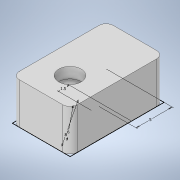
# Autodesk Inventor part: Bearing_Differential
Saved by Autodesk Inventor 2022.1 (Build 261234020, 234B)
## iProperties
Created: 2022-08-27
Part Number: Bearing_Differential
Material: Generic
Document SubType Name: Modeling
Designer: cdug029
Density: 1 g/cm^3
Appearance: Default
Author: cdug029
Autodesk Inventor part; units mm, degrees
ref_plane "YZ Plane" through (0, 0, 0) normal (1, 0, 0) x (0, 1, 0)
ref_plane "XZ Plane" through (0, 0, 0) normal (0, 1, 0) x (-1, 0, 0)
ref_plane "XY Plane" through (0, 0, 0) normal (0, 0, 1) x (1, 0, 0)
sketch "Sketch1" plane through (0, 0, 0) normal (0, 1, 0) x (-1, 0, 0)
  circle A0 centre (0, 0) radius 4 construction
  circle A1 centre (0, 0) radius 3 construction
  line L0 (-4.5, 4) -> (-4.5, -4) construction
  line L1 (4, -4) -> (-9, -4)
  line L2 (-9, -4) -> (-9, 4)
  line L3 (-9, 4) -> (4, 4)
  line L4 (4, 4) -> (4, -4)
  point P0 (-9, 0)
  dimension "d0" = 8
  dimension "d1" = 6
  dimension "d27" = 5
  dimension "d28" = 1.5
  constraints: 10 end point, 3 tangent, 2 centre point, 2 coincident, 2 parallel, 2 perpendicular, 2 point on line, 1 horizontal, 1 horizontal alignment
  measures "d0" diameter of A0
  measures "d1" diameter of A1
  measures "d27" distance edge to line of A0 L2
  measures "d28" distance edge to line of A1 L0
extrude "Extrusion1" add sketch "Sketch1" along normal blind 1.5
sketch "Sketch6" plane through (0, 1.5, 0) normal (0, 1, 0) x (1, 0, 0)
  circle A0 centre (0, 0) radius 1.55
  dimension "d29" = 3.1
  constraints: 1 centre point, 1 coincident
  measures "d29" diameter of A0
extrude "Extrusion6" cut sketch "Sketch6" against normal through all
sketch "Sketch7" plane through (0, 1.5, 0) normal (0, 1, 0) x (1, 0, 0)
  circle A0 centre (0, 0) radius 1.55 projected
  line L0 (-4, -4) -> (9, -4) projected
  line L1 (-4, 4) -> (-4, -4) projected
  line L2 (9, 4) -> (-4, 4) projected
  line L3 (9, -4) -> (9, 4) projected
  circle A1 centre (0, 0) radius 4 construction
  circle A2 centre (0, 0) radius 3 construction
  line L4 (-4, -4) -> (9, -4) projected
  line L5 (9, 4) -> (-4, 4) projected
  line L6 (4.5, 4) -> (4.5, -4)
  line L7 (-4, -4) -> (9, -4) projected
  dimension "d35" = 1.5
  constraints: 2 end point, 2 point on line, 1 perpendicular
  measures "d35" distance edge to line of A2 L6
extrude "Extrusion7" add sketch "Sketch7" along normal blind 1.35 contours A0 | L1 L2 L6 L0 | L6 L2 L3 L0
fillet "Fillet5" radius 1 4 edges at (-4, 1.425, 4) (9, 1.425, 4) (-4, 1.425, -4) (9, 1.425, -4)
mirror "Mirror2" about plane through (2.5, 2.85, 0) normal (0, 1, 0) of "Extrusion1", "Extrusion6", "Extrusion7", "Fillet5"
equation "\"d35\" = d28"
body "Solid1"
